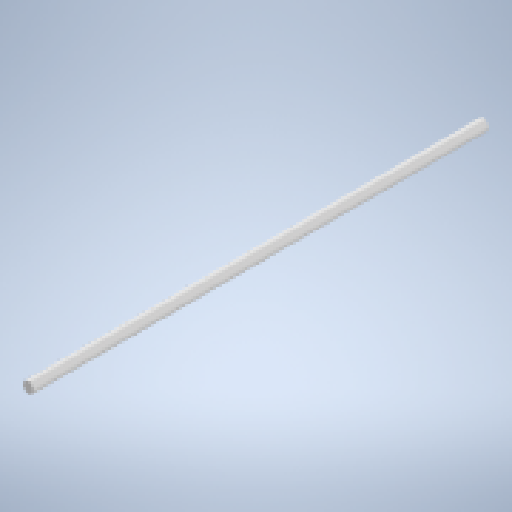
# Autodesk Inventor part: Axle1
Saved by Autodesk Inventor 2024 (Build 280153000, 153)
## iProperties
Created: 2024-04-11
Part Number: Axle1
Material: Iron, Gray
Document SubType Name: Modeling
Designer: teeta
Density: 7.15 g/cm^3
Appearance: Iron Gray
Author: teeta
Autodesk Inventor part; units mm, degrees
ref_plane "YZ Plane" through (0, 0, 0) normal (1, 0, 0) x (0, 1, 0)
ref_plane "XZ Plane" through (0, 0, 0) normal (0, 1, 0) x (-1, 0, 0)
sketch "Sketch1" plane through (0, 0, 0) normal (0, 0, 1) x (1, 0, 0)
  circle A0 centre (0, 0) radius 10.29 projected
  point P0 (0, 0)
ref_plane "Work Plane1" through (-12.0163, -12.0163, 844.8176) normal (0, 0, -1) x (-0.185, 0.9827, 0)
extrude "Extrusion1" add sketch "Sketch1" along normal up to surface (844.8176 mm away)
body "Solid1"
